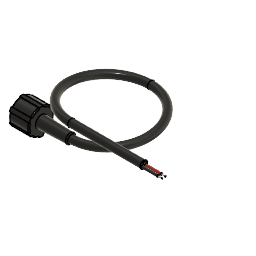
FA8 - 3-Pin Female Waterproof Connector (coiled) (Autodesk Fusion 360 design; units mm, degrees)
Autodesk Fusion 360 part; units mm, degrees
sketch "Sketch1" plane through (0, 0, 0) normal (1, 0, 0) x (0, 1, 0)
  circle A0 centre (0, 0) radius 6.35
  circle A1 centre (0, 0) radius 5.08
  dimension "d1" = 12.7
  dimension "d2" = 10.16
  constraint coincident A0.centre A1.centre
  constraint concentric A0 A1
  measures "d1" diameter of A0
  measures "d2" diameter of A1
extrude "Extrude1" add sketch "Sketch1" along normal blind 10 contours A0 | A1 makes body 1
extrude "Extrude2" cut sketch "Sketch1" along normal blind 8 contours A1 bodies 1
sketch "Sketch2" plane through (0, 0, 0) normal (0, 1, 0) x (1, 0, 0)
  line L0 (10, 0) -> (10, -3)
  line L1 (10, -3) -> (25, -2.5)
  line L2 (25, -2.5) -> (25, 0)
  line L3 (25, 0) -> (10, 0)
  dimension "d7" = 3
  constraint vertical L0
  constraint vertical L2
  constraint perpendicular L0 L3
  measures "d7" distance of L0.start L0.end
revolve "Revolve1" add sketch "Sketch2" angle 360 about axis through (1.75, 0, 0) along (1, 0, 0) bodies 1
fillet "Fillet1" radius 0.5 3 edges at (0, -5.9203, -2.2963) (10, -5.9203, -2.2963) (25, -0.904, -2.3308) on bodies 1
sketch "Sketch4" plane through (8, 0, 0) normal (1, 0, 0) x (0, 1, 0)
  line L0 (0, 1.5) -> (-1.299, -0.75) construction
  line L1 (-1.299, -0.75) -> (1.299, -0.75) construction
  line L2 (1.299, -0.75) -> (0, 1.5) construction
  circle A0 centre (0, 1.5) radius 0.5
  circle A1 centre (-1.299, -0.75) radius 0.5
  circle A2 centre (1.299, -0.75) radius 0.5
  circle A3 centre (0, 0) radius 2.25
  dimension "d15" = 1.5
  dimension "d16" = 1
  dimension "d17" = 1
  dimension "d18" = 1
  dimension "d43" = 4.5
  constraint coincident A3.centre origin
  constraint coincident L0.start L2.end
  constraint coincident L0.end L1.start
  constraint coincident L1.end L2.start
  measures "d15" distance of L0.start A3.centre
  measures "d16" diameter of A0
  measures "d17" diameter of A1
  measures "d18" diameter of A2
  measures "d43" diameter of A3
extrude "Extrude8" add sketch "Sketch4" against normal blind 8 bodies 1
sketch "Sketch10" plane through (0, 0, 0) normal (0, 0, 1) x (1, 0, 0)
  line L0 (10, -1) -> (0, -1)
  line L1 (0, 1) -> (10, 1)
  line L2 (10, 1) -> (10, -1)
  line L3 (10, -1) -> (0, 0) construction
  line L4 (0, 0) -> (10, 1) construction
  line L5 (0, -1) -> (0, 1)
  constraint horizontal L0
  constraint parallel L0 L1
  constraint coincident L3 L4.start
  constraint coincident L4 L3.end
  constraint coincident L3.end L4.start
extrude "Extrude9" add sketch "Sketch10" along normal blind 1 from surface at 5.5 bodies 1
pattern_circular "C-Pattern1" count 6 over 360 about axis through (1.75, 0, 0) along (1, 0, 0) of "Extrude9"
sketch "Sketch3" plane through (25, 0, 0) normal (1, 0, 0) x (0, 1, 0)
  circle A0 centre (0, 0) radius 1.905
  circle A1 centre (0, 0) radius 2.0164
  dimension "d9" = 3.81
  constraint coincident A0.centre A1.centre
  measures "d9" diameter of A0
sketch "Sketch5" plane through (0, 0, 0) normal (0, 0, 1) x (1, 0, 0)
  arc A0 through (25, 0, 0) (45, 19.9239, 1.7431) (25, 39.8478, 3.4862)
  arc A1 through (25, 39.8478, 3.4862) (5, 19.9239, 5.2293) (25, 0, 6.9725)
  dimension "d42" = 40
sweep "Sweep1" add profiles "Sketch3" path "Sketch5" along A0 A1 section 1 contours A0 bodies 1
extrude "Extrude5" add 1 faces at (25, -0.7992, 7.2336) along direction (1, 0, 0) blind 36.2 on bodies 1 bodies 1
sketch "Sketch6" plane through (61.2, 0, 0) normal (1, 0, 0) x (0, 1, 0)
  line L0 (0, 7.9725) -> (-0.866, 6.4725) construction
  line L1 (-0.866, 6.4725) -> (0.866, 6.4725) construction
  line L2 (0.866, 6.4725) -> (0, 7.9725) construction
  circle A0 centre (0, 7.9725) radius 0.625
  circle A1 centre (0.866, 6.4725) radius 0.625
  circle A2 centre (-0.866, 6.4725) radius 0.625
  circle A3 centre (0, 6.9725) radius 1.905
  point P0 (0, 6.9725)
  dimension "d31" = 1
  dimension "d32" = 1.25
  dimension "d33" = 1.25
  dimension "d34" = 1.25
  constraint coincident L0.start L2.end
  constraint coincident L1.end L2.start
  constraint coincident L0.end L1.start
  measures "d31" distance of L0.start P0
  measures "d32" diameter of A0
  measures "d33" diameter of A1
  measures "d34" diameter of A2
extrude "Extrude6" add sketch "Sketch6" along normal blind 8 separate body contours A1 | A2 makes body 2 at (63.8667, -0.2441, 6.4102) makes body 3 at (63.8667, 1.4879, 6.4102)
sketch "Sketch7" plane through (69.2, 0, 0) normal (1, 0, 0) x (0, 1, 0)
  circle A0 centre (0, 7.9725) radius 0.375
  circle A1 centre (0.866, 6.4725) radius 0.625
  circle A2 centre (-0.866, 6.4725) radius 0.625
  dimension "d52" = 0.75
  measures "d52" diameter of A0
sketch "Sketch8" plane through (69.2, 0, 0) normal (1, 0, 0) x (0, 1, 0)
  circle A0 centre (0.866, 6.4725) radius 0.625
  circle A1 centre (0.866, 6.4725) radius 0.375
  dimension "d37" = 0.75
  constraint concentric A0 A1
  measures "d37" diameter of A1
sketch "Sketch9" plane through (69.2, 0, 0) normal (1, 0, 0) x (0, 1, 0)
  circle A0 centre (-0.866, 6.4725) radius 0.625
  circle A1 centre (-0.866, 6.4725) radius 0.375
  dimension "d38" = 0.75
  constraint concentric A0 A1
  measures "d38" diameter of A1
extrude "Extrude7" add sketch "Sketch8" sketch "Sketch9" along normal blind 2 separate body contours A1 of sketch 2 contours A1 makes body 4 at (69.8667, 1.2392, 6.4351) makes body 5 at (69.8667, -0.4929, 6.4351)
extrude "Extrude10" add sketch "Sketch6" along normal blind 0.5 separate body contours A0 makes body 6
